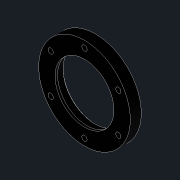
# Autodesk Inventor part: unit-base1
Saved by Autodesk Inventor 2022 (Build 260153000, 153)
## iProperties
Created: 2021-07-12
Part Number: unit-base1
Material: ABS プラスチック
Document SubType Name: Modeling
Designer: yuta0
Density: 1.06 g/cm^3
Appearance: 滑らか - 黒
Mass: 21.8509 g
Surface Area: 94.5687 cm^2
Volume: 20.6141 cm^3
購入先: 印刷
在庫数: 0.0
Author: yuta0
Autodesk Inventor part; units mm, degrees
ref_plane "YZ Plane" through (0, 0, 0) normal (1, 0, 0) x (0, 1, 0)
ref_plane "XZ Plane" through (0, 0, 0) normal (0, 1, 0) x (-1, 0, 0)
ref_plane "XY Plane" through (0, 0, 0) normal (0, 0, 1) x (1, 0, 0)
sketch "スケッチ1" plane through (0, 0, 0) normal (1, 0, 0) x (0, 1, 0)
  line L0 (24.1, 0) -> (24.1, -2)
  line L1 (24.1, -2) -> (26.1, -2)
  line L2 (26.1, -2) -> (26.1, -9)
  line L3 (26.1, -9) -> (37.5, -9)
  line L4 (37.5, -9) -> (37.5, 0)
  line L5 (37.5, 0) -> (24.1, 0)
  line L6 (0, -10.8) -> (0, 1.8) projected
  point P0 (0, 0)
  dimension "d0" = 26.1
  dimension "d1" = 37.5
  dimension "d2" = 7
  dimension "d3" = 2
  dimension "d4" = 2
  constraints: 12 end point, 5 perpendicular, 1 horizontal alignment, 1 vertical
  measures "d0" distance from line of point (0, 0) L2
  measures "d1" distance from line of point (0, 0) L4
  measures "d2" distance of L1.end L2.end
  measures "d3" distance of L0.start L0.end
  measures "d4" distance of L0.end L1.end
revolve "回転1" add sketch "スケッチ1" angle 360 about axis through (0, 0, -10) along (0, 0, 1)
sketch "スケッチ2" plane through (0, 0, -9) normal (0, 0, -1) x (-1, 0, 0)
  circle A0 centre (0, 0) radius 32
  point P0 (0, 32)
  point P1 (-27.7128, 16)
  point P2 (-27.7128, -16)
  point P3 (0, -32)
  point P4 (27.7128, -16)
  point P5 (27.7128, 16)
  dimension "d6" = 64
  dimension "d9" = 360
  constraints: 2 vertical alignment, 1 coincident, 9 other
hole "穴1" at (0, 32, -9) at (27.7128, 16, -9) at (27.7128, -16, -9) at (0, -32, -9) at (-27.7128, -16, -9) at (-27.7128, 16, -9) direction (0, 0, 1) diameter 4.3 end through all clearance for "Socket Head Cap Screw" size "M4" standard "Ansi Metric M Profile"
chamfer "面取り1" distance 0.5 angle 45 1 edges at (0, -26.1, -9)
sketch "スケッチ3" plane through (0, 0, -9) normal (0, 0, -1) x (-1, 0, 0)
  circle A0 centre (-37.5, 0) radius 4.8
  circle A1 centre (0, 0) radius 37.5 projected
  point P0 (-37.1928, 4.7902)
  point P1 (-37.1928, -4.7902)
  dimension "d18" = 9.6
  constraints: 1 centre point, 1 horizontal alignment, 2 other
  measures "d18" diameter of A0
